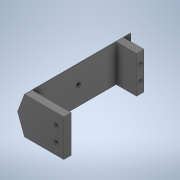
# Autodesk Inventor part: BodyWedgeSideV3.1
Saved by Autodesk Inventor 2020 (Build 240168000, 168)
## iProperties
Created: 2023-12-06
Part Number: BodyWedgeSideV3.1
Material: Thermoplastic Resin
Document SubType Name: Modeling
Designer: smz3rm
Density: 1.28 g/cm^3
Appearance: Smooth - Black
Mass: 23.6548 g
Surface Area: 81.6035 cm^2
Volume: 18.4803 cm^3
Author: smz3rm
Autodesk Inventor part; units mm, degrees
ref_plane "YZ Plane" through (0, 0, 0) normal (1, 0, 0) x (0, 1, 0)
ref_plane "XZ Plane" through (0, 0, 0) normal (0, 1, 0) x (-1, 0, 0)
sketch "Sketch1" plane through (0, 0, 0) normal (0, 0, 1) x (1, 0, 0)
  line L0 (0, -21) -> (0, 21) projected
  line L1 (0, 15) -> (0, -15)
  line L2 (0, -15) -> (-0.4, -15)
  line L3 (-0.4, -15) -> (-15, 0)
  line L4 (-15, 0) -> (-0.4, 15)
  line L5 (-0.4, 15) -> (0, 15)
  point P0 (0, 0)
  point P1 (0, 0)
  dimension "d1" = 30
  dimension "d5" = 15
  dimension "d50" = 0.4
  dimension "d51" = 15
  constraints: 10 end point, 2 equal length, 2 midpoint, 2 point on line, 1 horizontal, 1 perpendicular, 1 vertical
  measures "d1" distance of L1.end L1.start
  measures "d5" distance of L1.end point (0, 0)
  measures "d50" distance of L1.end L2.end
  measures "d51" distance from line of L0 L3.end
ref_plane "Work Plane1" through (0, 0, 86) normal (0, 0, 1) x (1, 0, 0)
sketch "Sketch2" plane through (0, 0, 86) normal (0, 0, 1) x (1, 0, 0)
  line L0 (0, -21) -> (0, 21) projected
  line L1 (0, 15) -> (0, -15)
  line L2 (0, -15) -> (-0.4, -15)
  line L3 (-0.4, -15) -> (-6, 0)
  line L4 (-6, 0) -> (-0.4, 15)
  line L5 (-0.4, 15) -> (0, 15)
  point P0 (0, 0)
  dimension "d3" = 30
  dimension "d6" = 15
  dimension "d52" = 0.4
  dimension "d53" = 6
  constraints: 10 end point, 2 equal length, 2 point on line, 1 horizontal, 1 parallel
  measures "d3" distance of L1.start L1.end
  measures "d6" distance of point (0, 0) L1.end
  measures "d52" distance of L1.end L2.end
  measures "d53" distance from line of L3.end L0
loft "Loft1" add profiles "Sketch2", "Sketch1"
sketch "Sketch3" plane through (0, -15, 86) normal (1, 0, 0) x (0, 0, -1)
  line L0 (0, 30) -> (86, 30) projected
  line L1 (0, 0) -> (86, 0) projected
  line L2 (0, 30) -> (6, 30)
  line L3 (6, 30) -> (6, 0)
  line L4 (6, 0) -> (0, 0)
  line L5 (0, 0) -> (0, 30)
  line L6 (74, 30) -> (80, 30)
  line L7 (80, 30) -> (80, 0)
  line L8 (80, 0) -> (74, 0)
  line L9 (74, 0) -> (74, 30)
  point P0 (86, 15)
  point P1 (74, 0)
  dimension "d11" = 6
  dimension "d12" = 6
  dimension "d13" = 6
  constraints: 16 end point, 4 parallel, 3 point on line, 2 horizontal, 2 perpendicular
  measures "d11" distance of L0.start L2.end
  measures "d12" distance of L6.end L6.start
  measures "d13" distance of L6.end L0.end
extrude "Extrusion1" add sketch "Sketch3" along normal blind 16.51 contours L0 L3 L1 L5 | L0 L7 L1 L9
sketch "Sketch4" plane through (0, -15, 80) normal (1, 0, 0) x (0, 0, -1)
  circle A0 centre (37.25, 15) radius 1.75
  line L0 (-6, 30) -> (-6, 0) projected
  line L1 (-6, 15) -> (80, 15) projected
  dimension "d16" = 43.25
  dimension "d17" = 3.5
  constraints: 1 centre point, 1 point on line
  measures "d16" distance from line of L0 A0.centre
  measures "d17" diameter of A0
extrude "Extrusion2" cut sketch "Sketch4" against normal through all
sketch "Sketch5" plane through (0, -15, 0) normal (0, 0, -1) x (-1, 0, 0)
  line L0 (0, 0) -> (0, 30) projected
  circle A0 centre (6.2132, 15) radius 6.2132
  line L1 (15, 15) -> (0, 0) projected
  line L2 (0, 30) -> (15, 15) projected
  line L3 (0, 0) -> (0, 30) projected
  circle A1 centre (6.2132, 15) radius 1.75
  line L4 (0.4, 30) -> (15, 15) projected
  line L5 (0, 30) -> (0.4, 30) projected
  line L6 (0.4, 0) -> (0, 0) projected
  line L7 (15, 15) -> (0.4, 0) projected
  point P0 (0, 15)
  dimension "d20" = 3.5
  constraints: 3 tangent, 2 centre point, 1 coincident
  measures "d20" diameter of A1
extrude "Extrusion3" add sketch "Sketch5" along normal blind 3 contours A1
sketch "Sketch6" plane through (16.51, -15, 86) normal (1, 0, 0) x (0, 0, -1)
  line L0 (6, 0) -> (6, 30) projected
  line L1 (6, 30) -> (0, 30) projected
  line L2 (0, 30) -> (0, 0) projected
  line L3 (0, 0) -> (6, 0) projected
  point P0 (86, 15)
extrude "Extrusion4" add sketch "Sketch6" along normal blind 12
sketch "Sketch8" plane through (16.51, -15, 86) normal (1, 0, 0) x (0, 0, -1)
  line L0 (74, 3) -> (80, 3)
  line L1 (74, 0) -> (80, 0) projected
  line L2 (74, 27) -> (80, 27)
  line L3 (80, 30) -> (74, 30) projected
  line L4 (74, 0) -> (74, 30) projected
  line L5 (74, 21) -> (80, 21)
  line L6 (74, 9) -> (80, 9)
  circle A0 centre (77, 21) radius 1.45
  circle A1 centre (77, 9) radius 1.45
  line L7 (80, 0) -> (80, 30) projected
  point P0 (86, 15)
  dimension "d25" = 3
  dimension "d26" = 3
  dimension "d27" = 6
  dimension "d28" = 6
  dimension "d29" = 2.9
  dimension "d30" = 2.9
  dimension "d48" = 3
  dimension "d49" = 3
  constraints: 8 end point, 4 horizontal, 2 centre point, 2 midpoint, 2 point on line
  measures "d25" distance between parallel lines of L1 L0
  measures "d26" distance between parallel lines of L2 L3
  measures "d27" distance between parallel lines of L0 L6
  measures "d28" distance between parallel lines of L2 L5
  measures "d29" diameter of A0
  measures "d30" diameter of A1
  measures "d48" distance from line of L7 A0.centre
  measures "d49" distance from line of L7 A1.centre
extrude "Extrusion5" cut sketch "Sketch8" against normal blind 7 contours A1 L6 | L6 A1 | A0 L5 | L5 A0
sketch "Sketch9" plane through (0, -15, 86) normal (0, 0, 1) x (1, 0, 0)
  line L0 (0, 30) -> (28.51, 30) projected
  line L1 (22.51, 30) -> (22.51, 0.0044)
  line L2 (28.51, 30) -> (28.51, 0) projected
  line L3 (28.51, 30) -> (0, 30) projected
  line L4 (-0.4, 0) -> (28.51, 0) projected
  line L5 (28.51, 3) -> (0.1043, 3)
  line L6 (28.51, 27) -> (0.4735, 27)
  line L7 (25.51, 30) -> (25.51, 0)
  line L8 (22.51, 21) -> (28.51, 21)
  line L9 (28.51, 0) -> (28.51, 30) projected
  line L10 (22.51, 9) -> (28.51, 9)
  circle A0 centre (25.51, 21) radius 1.45
  circle A1 centre (25.51, 9) radius 1.45
  point P0 (0, 15)
  point P1 (16.51, 0)
  point P2 (16.51, 30)
  point P3 (0, 0)
  dimension "d33" = 6
  dimension "d35" = 3
  dimension "d36" = 3
  dimension "d43" = 3
  dimension "d44" = 6
  dimension "d45" = 6
  dimension "d46" = 2.9
  dimension "d47" = 2.9
  constraints: 12 end point, 9 point on line, 4 horizontal, 2 centre point, 2 midpoint, 1 perpendicular, 1 vertical
  measures "d33" distance between parallel lines of L2 L1
  measures "d35" distance of L2.end L5.start
  measures "d36" distance of L0.end L6.start
  measures "d43" distance of L0.end L7.start
  measures "d44" distance between parallel lines of L6 L8
  measures "d45" distance between parallel lines of L5 L10
  measures "d46" diameter of A0
  measures "d47" diameter of A1
extrude "Extrusion6" cut sketch "Sketch9" against normal up to surface (6 mm away) contours A0 L8 L7 | L7 L8 A0 | L8 L7 A0 | L8 A0 L7 | A1 L7 L10 | L10 L7 A1 | L10 A1 L7 | L7 A1 L10
sketch "Sketch10" plane through (28.51, -15, 86) normal (1, 0, 0) x (0, 0, -1)
  line L0 (6, 30) -> (0, 30) projected
  line L1 (0, 30) -> (0, 0) projected
  line L2 (0, 0) -> (6, 0) projected
  line L3 (6, 0) -> (6, 30) projected
  point P0 (86, 15)
extrude "Extrusion7" add sketch "Sketch10" along normal blind 3
equation "\"d1\" = Height"
equation "\"d5\" = 0.5 * Height"
equation "\"d51\" = SideArmorWidth"
equation "\"d3\" = Height"
equation "\"d6\" = 0.5 * Height"
equation "\"d53\" = SideThickness"
equation "\"d11\" = SideThickness"
equation "\"d12\" = SideThickness"
equation "\"d13\" = SideThickness"
equation "\"d14\" = WheelWidth"
equation "\"d16\" = DriveMotorOffset + SideThickness"
equation "\"d17\" = DriveMotorHoleDia"
equation "\"d20\" = ForkPlugDia"
equation "\"d21\" = ForkPlugLength"
equation "\"d23\" = 2 * SideThickness"
equation "\"d25\" = BaseThickness"
equation "\"d26\" = BaseThickness"
equation "\"d27\" = SideThickness"
equation "\"d28\" = SideThickness"
equation "\"d29\" = ScrewDia"
equation "\"d30\" = ScrewDia"
equation "\"d48\" = 0.5 * SideThickness"
equation "\"d49\" = 0.5 * SideThickness"
equation "\"d31\" = ScrewDepth"
equation "\"d33\" = SideThickness"
equation "\"d35\" = BaseThickness"
equation "\"d36\" = BaseThickness"
equation "\"d43\" = 0.5 * SideThickness"
equation "\"d44\" = SideThickness"
equation "\"d45\" = SideThickness"
equation "\"d46\" = ScrewDia"
equation "\"d47\" = ScrewDia"
equation "\"d2\" = BoxLength + SideThickness"
equation "\"Height\" = 30"
equation "\"SideArmorWidth\" = 15"
equation "\"SideThickness\" = 6"
equation "\"WheelWidth\" = 16.51"
equation "\"DriveMotorOffset\" = 37.25"
equation "\"DriveMotorHoleDia\" = 3.5"
equation "\"ForkPlugDia\" = 3.5"
equation "\"ForkPlugLength\" = 3"
equation "\"BaseThickness\" = 3"
equation "\"ScrewDia\" = 2.9"
equation "\"ScrewDepth\" = 7"
equation "\"BoxLength\" = 80"
body "Solid1"
